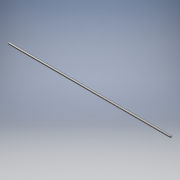
# Autodesk Inventor part: Main Axle
Saved by Autodesk Inventor 2019.4 (Build 234330000, 330)
## iProperties
Created: 2020-01-05
Part Number: Main Axle
Material: Steel, Mild
Document SubType Name: Modeling
Designer: admin
Density: 7.85 g/cm^3
Appearance: Semi-Polished
Author: admin
Autodesk Inventor part; units mm, degrees
ref_plane "YZ Plane" through (0, 0, 0) normal (1, 0, 0) x (0, 1, 0)
ref_plane "XZ Plane" through (0, 0, 0) normal (0, 1, 0) x (-1, 0, 0)
ref_plane "XY Plane" through (0, 0, 0) normal (0, 0, 1) x (1, 0, 0)
sketch "Sketch1" plane through (0, 0, 0) normal (0, 0, 1) x (1, 0, 0)
  line L0 (0, 0) -> (0, 5)
  line L1 (800, 5) -> (800, 0)
  line L2 (800, 0) -> (0, 0)
  line L3 (0, 5) -> (2, 5)
  line L4 (2, 5) -> (2, 4.65)
  line L5 (2, 4.65) -> (3.1, 4.65)
  line L6 (3.1, 4.65) -> (3.1, 5)
  line L7 (3.1, 5) -> (24.6, 5)
  line L8 (24.6, 5) -> (24.6, 4.65)
  line L9 (24.6, 4.65) -> (25.7, 4.65)
  line L10 (25.7, 4.65) -> (25.7, 5)
  line L11 (25.7, 5) -> (793.9, 5)
  line L12 (793.9, 5) -> (793.9, 4.65)
  line L13 (793.9, 4.65) -> (795, 4.65)
  line L14 (795, 4.65) -> (795, 5)
  line L15 (795, 5) -> (800, 5)
  dimension "d0" = 5
  dimension "d4" = 800
  dimension "d6" = 0.35
  dimension "d7" = 1.1
  dimension "d8" = 2
  dimension "d9" = 0.35
  dimension "d10" = 1.1
  dimension "d11" = 21.5
  dimension "d12" = 0.35
  dimension "d13" = 1.1
  dimension "d14" = 5
  constraints: 32 end point, 10 perpendicular, 4 point on line, 3 horizontal, 2 vertical
  measures "d0" distance of L0.start L0.end
  measures "d4" distance of L0.end L1.start
  measures "d6" distance of L3.end L4.end
  measures "d7" distance of L4.end L5.end
  measures "d8" distance of L0.end L3.end
  measures "d9" distance of L7.end L8.end
  measures "d10" distance of L8.end L9.end
  measures "d11" distance of L6.end L7.end
  measures "d12" distance of L11.end L12.end
  measures "d13" distance of L12.end L13.end
  measures "d14" distance between parallel lines of L1 L14
revolve "Revolution1" add sketch "Sketch1" angle 360 about axis through (800, 0, 0) along (-1, 0, 0)
body "Solid1"
